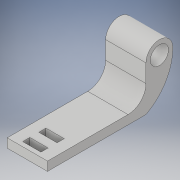
# Autodesk Inventor part: WheelIntakeBase3.0
Saved by Autodesk Inventor 2017 (Build 210142000, 142)
## iProperties
Created: 2017-12-09
Part Number: WheelIntakeBase3.0
Material: Generic
Document SubType Name: Modeling
Designer: User
Density: 1 g/cm^3
Appearance: Default
Author: User
Autodesk Inventor part; units mm, degrees
ref_plane "YZ Plane" through (0, 0, 0) normal (1, 0, 0) x (0, 1, 0)
ref_plane "XZ Plane" through (0, 0, 0) normal (0, 1, 0) x (-1, 0, 0)
ref_plane "XY Plane" through (0, 0, 0) normal (0, 0, 1) x (1, 0, 0)
sketch "Sketch1" plane through (0, 0, 0) normal (1, 0, 0) x (0, 1, 0)
  circle A0 centre (0, 0) radius 9.525
  line L0 (0, 9.525) -> (-25.4, 9.525)
  line L1 (-31.75, 9.525) -> (-31.75, 79.375)
  line L2 (-31.75, 79.375) -> (-25.4, 79.375)
  line L3 (-25.4, 79.375) -> (-25.4, 9.525)
  arc A1 (-31.75, 9.525) -> (0.0899, -9.5246) centre (-0.2457, 26.0482) ccw
  dimension "d0" = 19.05
  dimension "d4" = 25.4
  dimension "d5" = 69.85
  dimension "d6" = 6.35
  constraints: 8 end point, 4 point on circle, 2 centre point, 1 coincident, 1 horizontal, 1 parallel, 1 tangent
  measures "d0" diameter of A0
  measures "d4" distance of L0.start L0.end
  measures "d5" distance of L2.end L0.end
  measures "d6" distance of L1.end L2.end
extrude "Extrusion1" add sketch "Sketch1" along normal blind 28.575
fillet "Fillet1" radius 12.7 1 edges at (14.2875, -25.4, 9.525)
sketch "Sketch2" plane through (28.575, 0, 0) normal (1, 0, 0) x (0, 0, -1)
  line L0 (-9.525, 0) -> (-9.525, -12.7) projected
  arc A0 (-22.225, -25.4) -> (-9.525, -12.7) centre (-22.225, -12.7) ccw projected
  line L1 (-22.225, -25.4) -> (-79.375, -25.4) projected
  line L2 (-79.375, -25.4) -> (-79.375, -31.75) projected
  line L3 (-79.375, -31.75) -> (-9.525, -31.75) projected
  arc A1 (-9.525, -31.75) -> (9.5246, 0.0899) centre (-26.0482, -0.2457) ccw projected
  arc A2 (9.5246, 0.0899) -> (-9.525, 0) centre (0, 0) ccw projected
hole "Hole1" at (28.575, 0, 0) direction (-1, 0, 0) diameter 12.827 depth 25.4 tip angle 118
sketch "Sketch3" plane through (0, -25.4, 79.375) normal (0, 1, 0) x (1, 0, 0)
  line L0 (0, 57.15) -> (28.575, 57.15) projected
  line L1 (0, 57.15) -> (0, 0) projected
  line L2 (0, 0) -> (28.575, 0) projected
  line L3 (28.575, 57.15) -> (28.575, 0) projected
  line L4 (7.8105, 3.175) -> (20.7645, 3.175)
  line L5 (20.7645, 3.175) -> (20.7645, 8.255)
  line L6 (20.7645, 8.255) -> (7.8105, 8.255)
  line L7 (7.8105, 8.255) -> (7.8105, 3.175)
  line L8 (7.8105, 19.685) -> (20.7645, 19.685)
  line L9 (20.7645, 19.685) -> (20.7645, 14.605)
  line L10 (20.7645, 14.605) -> (7.8105, 14.605)
  line L11 (7.8105, 14.605) -> (7.8105, 19.685)
  point P0 (0, 79.375)
  dimension "d17" = 12.954
  dimension "d18" = 5.08
  dimension "d19" = 7.8105
  dimension "d20" = 28.575
  dimension "d21" = 3.175
  dimension "d22" = 5.08
  dimension "d23" = 6.35
  dimension "d24" = 12.954
  constraints: 16 end point, 4 parallel, 2 horizontal, 2 perpendicular
  measures "d17" distance of L6.end L5.end
  measures "d18" distance of L5.end L4.end
  measures "d19" distance between parallel lines of L1 L7
  measures "d20" distance of L1.end L2.end
  measures "d21" distance between parallel lines of L2 L4
  measures "d22" distance of L8.end L9.end
  measures "d23" distance between parallel lines of L6 L10
  measures "d24" distance of L8.start L8.end
extrude "Extrusion2" cut sketch "Sketch3" against normal blind 25.4 contours L7 L6 L5 L4 | L8 L9 L10 L11
equation "\"d19\" = -0.5 * d17 + 0.5 * d20"
body "Solid1"
